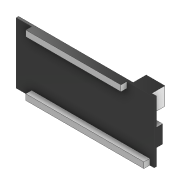
# Autodesk Inventor part: Dummy_ESP32_LOLIN_D32
Saved by Autodesk Inventor 2020 (Build 240168000, 168)
## iProperties
Created: 2020-10-27
Part Number: Dummy_ESP32_LOLIN_D32
Material: Generisch
Document SubType Name: Modeling
Designer: uhlma
Density: 1 g/cm^3
Appearance: Vorgabe
Author: uhlma
Autodesk Inventor part; units mm, degrees
ref_plane "YZ Plane" through (0, 0, 0) normal (1, 0, 0) x (0, 1, 0)
ref_plane "XZ Plane" through (0, 0, 0) normal (0, 1, 0) x (-1, 0, 0)
ref_plane "Arbeitsebene1" through (0, 0, 0) normal (0, 0, -1) x (-1, 0, 0)
sketch "Skizze5" plane through (0, 0, 0) normal (0, 0, -1) x (-1, 0, 0)
  line L0 (29.5, 13.05) -> (-29.5, 13.05)
  line L1 (-29.5, 13.05) -> (-29.5, -13.05)
  line L2 (-29.5, -13.05) -> (29.5, -13.05)
  line L3 (29.5, -13.05) -> (29.5, 13.05)
  point P0 (0, 0)
  point P1 (29.5, 0)
  point P2 (0, -13.05)
  dimension "d70" = 26.1
  dimension "d71" = 59
  constraints: 8 end point, 2 midpoint, 2 parallel, 1 horizontal, 1 horizontal alignment, 1 perpendicular, 1 vertical alignment
  measures "d70" distance of L2.end L0.start
  measures "d71" distance of L1.end L2.end
extrude "Extrusion5" add sketch "Skizze5" along normal blind 1
sketch "Skizze4" plane through (0, 0, 0) normal (0, 0, -1) x (-1, 0, 0)
  line L0 (22.9, 13.05) -> (-17.8, 13.05)
  line L1 (-17.8, 13.05) -> (-17.8, 10.55)
  line L2 (-17.8, 10.55) -> (22.9, 10.55)
  line L3 (22.9, 10.55) -> (22.9, 13.05)
  line L4 (29.5, -13.05) -> (29.5, 13.05) projected
  line L5 (-29.5, -13.05) -> (29.5, -13.05) projected
  line L6 (29.5, 13.05) -> (-29.5, 13.05) projected
  line L7 (22.9, -13.05) -> (-27.6, -13.05)
  line L8 (-27.6, -13.05) -> (-27.6, -10.55)
  line L9 (-27.6, -10.55) -> (22.9, -10.55)
  line L10 (22.9, -10.55) -> (22.9, -13.05)
  dimension "d68" = 40.7
  dimension "d69" = 2.5
  dimension "d77" = 6.6
  dimension "d78" = 50.5
  constraints: 16 end point, 4 parallel, 2 collinear, 2 horizontal, 2 perpendicular, 1 point on line, 1 vertical alignment
  measures "d68" distance from line of L1.end L3
  measures "d69" distance between parallel lines of L2 L0
  measures "d77" distance between parallel lines of L3 L4
  measures "d78" distance from line of L7.start L8
extrude "Extrusion4" add sketch "Skizze4" against normal blind 2.5
sketch "Skizze6" plane through (0, 0, -1) normal (0, 0, -1) x (-1, 0, 0)
  line L0 (22.2, -9) -> (4.2, -9)
  line L1 (4.2, -9) -> (4.2, 9)
  line L2 (4.2, 9) -> (22.2, 9)
  line L3 (22.2, 9) -> (22.2, -9)
  line L4 (29.5, -13.05) -> (29.5, 13.05) projected
  point P0 (0, 0)
  point P1 (4.2, 0)
  dimension "d26" = 18
  dimension "d27" = 18
  dimension "d72" = 7.3
  constraints: 8 end point, 2 parallel, 1 horizontal, 1 horizontal alignment, 1 midpoint, 1 perpendicular
  measures "d26" distance between parallel lines of L1 L3
  measures "d27" distance between parallel lines of L2 L0
  measures "d72" distance between parallel lines of L4 L3
extrude "Extrusion6" add sketch "Skizze6" along normal blind 3.2
sketch "Skizze7" plane through (0, 0, -1) normal (0, 0, -1) x (-1, 0, 0)
  line L0 (-24.3, -6.05) -> (-29.5, -6.05)
  line L1 (-29.5, -6.05) -> (-29.5, 1.45)
  line L2 (-29.5, 1.45) -> (-24.3, 1.45)
  line L3 (-24.3, 1.45) -> (-24.3, -6.05)
  line L4 (-29.5, 13.05) -> (-29.5, -13.05) projected
  line L5 (-29.5, -13.05) -> (29.5, -13.05) projected
  point P0 (0, 0)
  dimension "d31" = 7.5
  dimension "d32" = 5.2
  dimension "d73" = 7
  dimension "d74" = 0
  constraints: 8 end point, 2 parallel, 1 horizontal, 1 perpendicular
  measures "d31" distance between parallel lines of L0 L2
  measures "d32" distance between parallel lines of L1 L3
  measures "d73" distance between parallel lines of L5 L0
  measures "d74" distance between parallel lines of L1 L4
extrude "Extrusion7" add sketch "Skizze7" along normal blind 2.6
sketch "Skizze8" plane through (0, 0, -1) normal (0, 0, -1) x (-1, 0, 0)
  line L0 (-19.5, 5.45) -> (-27.5, 5.45)
  line L1 (-27.5, 5.45) -> (-27.5, 13.05)
  line L2 (-27.5, 13.05) -> (-19.5, 13.05)
  line L3 (-19.5, 13.05) -> (-19.5, 5.45)
  line L4 (29.5, 13.05) -> (-29.5, 13.05) projected
  line L5 (-29.5, 13.05) -> (-29.5, 1.45) projected
  point P0 (0, 0)
  dimension "d36" = 7.6
  dimension "d37" = 8
  dimension "d75" = 0
  dimension "d79" = 2
  constraints: 8 end point, 2 parallel, 1 horizontal, 1 perpendicular
  measures "d36" distance between parallel lines of L2 L0
  measures "d37" distance between parallel lines of L1 L3
  measures "d75" distance between parallel lines of L4 L2
  measures "d79" distance between parallel lines of L5 L1
extrude "Extrusion8" add sketch "Skizze8" along normal blind 5.6
